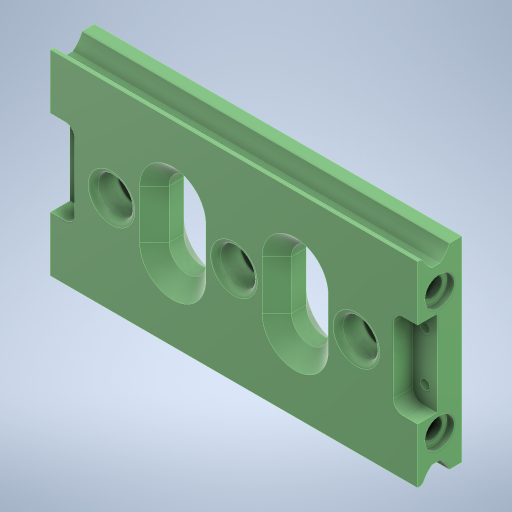
# Autodesk Inventor part: Rail-150MM
Saved by Autodesk Inventor 2023.1 (Build 271208000, 208)
## iProperties
Created: 2023-06-05
Part Number: Rail-150MM
Material: ABS Plastic
Document SubType Name: Modeling
Designer: hello
Density: 1.06 g/cm^3
Appearance: Smooth - Dark Forest Green
Mass: 267.479 g
Surface Area: 701.462 cm^2
Volume: 252.338 cm^3
Author: hello
Autodesk Inventor part; units mm, degrees
ref_plane "YZ Plane" through (0, 0, 0) normal (1, 0, 0) x (0, 1, 0)
ref_plane "XZ Plane" through (0, 0, 0) normal (0, 1, 0) x (-1, 0, 0)
ref_plane "XY Plane" through (0, 0, 0) normal (0, 0, 1) x (1, 0, 0)
sketch "Sketch1" plane through (0, 0, 0) normal (1, 0, 0) x (0, 1, 0)
  line L0 (-40, 0) -> (40, 0)
  line L1 (-40, 0) -> (-40, 5)
  line L2 (40, 0) -> (40, 5)
  line L3 (-40, 16) -> (-40, 18)
  line L4 (-40, 18) -> (40, 18)
  line L5 (40, 18) -> (40, 16)
  line L6 (0, 0) -> (0, 18) construction
  line L7 (-25, 9) -> (25, 9) construction
  circle A0 centre (-25, 9) radius 4.025
  circle A1 centre (25, 9) radius 4.025
  circle A2 centre (-40.25, 10.5) radius 5 construction
  arc A3 (-33.7571, 10.5) -> (-40, 16) centre (-44.3193, 4.8043) ccw
  arc A4 (-40, 5) -> (-33.7571, 10.5) centre (-44.3193, 16.1957) ccw
  line L8 (-40, 16) -> (-40, 5) construction
  arc A5 (40, 16) -> (33.7571, 10.5) centre (44.3193, 4.8043) ccw
  arc A6 (33.7571, 10.5) -> (40, 5) centre (44.3193, 16.1957) ccw
  line L9 (-34.8, 12.1107) -> (-34.8, 8.8893)
  line L10 (34.8, 12.1107) -> (34.8, 8.8893)
  point P0 (0, 9)
  point P1 (-40, 10.5)
  point P2 (-34.8, 10.5)
  dimension "d0" = 80
  dimension "d6" = 2
  dimension "d9" = 18
  dimension "d10" = 50
  dimension "d11" = 8.05
  dimension "d12" = 8.05
  dimension "d60" = 5
  dimension "d61" = 10
  dimension "d62" = 12
  dimension "d63" = 6.2429
  dimension "d64" = 0.25
  dimension "d65" = 12
  dimension "d66" = 12
  dimension "d67" = 6.2429
  dimension "d68" = 5.2
  constraints: 22 end point, 12 point on circle, 7 centre point, 6 midpoint, 5 horizontal alignment, 4 vertical, 3 coincident, 2 horizontal, 2 parallel, 2 tangent, 2 vertical alignment, 1 collinear, 1 equal radius, 1 perpendicular
  measures "d0" distance of L0.start L0.end
  measures "d6" distance of L3.start L3.end
  measures "d9" distance of L6.start L6.end
  measures "d10" distance of L7.start L7.end
  measures "d11" diameter of A0
  measures "d12" diameter of A1
  measures "d60" distance of L0.start L1.end
  measures "d61" diameter of A2
  measures "d62" radius of A3
  measures "d63" distance from line of A3.start L1
  measures "d64" distance of point (-40, 10.5) A2.centre
  measures "d65" radius of A5
  measures "d66" radius of A6
  measures "d67" distance from line of A5.end L2
  measures "d68" distance from line of point (-34.8, 10.5) L3
extrude "Extrusion1" add sketch "Sketch1" along normal blind 150
sketch "Sketch3" plane through (0, -40, 18) normal (0, 0, 1) x (1, 0, 0)
  line L0 (0, 80) -> (0, 0) projected
  point P0 (0, 40)
  point P1 (25, 40)
  point P2 (0, 40)
  point P3 (0, 40)
  dimension "d13" = 25
  constraints: 2 midpoint, 1 horizontal alignment
  measures "d13" distance of point (25, 40) point (0, 40)
hole "Hole1" at (25, 0, 18) direction (0, 0, -1) diameter 5.5 end through all counterbore diameter 15 counterbore depth 10 clearance for "Hex Head Cap Screw DIN EN 24017" size "M5" standard "DIN"
pattern_linear "Rectangular Pattern1" count 3 spacing 50 along (1, 0, 0) of "Hole1"
sketch "Sketch4" plane through (0, -40, 18) normal (0, 0, 1) x (1, 0, 0)
  line L0 (0, 57.5) -> (6, 57.5)
  line L1 (10, 53.5) -> (10, 26.5)
  line L2 (6, 22.5) -> (0, 22.5)
  line L3 (0, 22.5) -> (0, 57.5)
  line L4 (0, 80) -> (0, 0) construction
  arc A0 (10, 53.5) -> (6, 57.5) centre (6, 53.5) ccw
  arc A1 (6, 22.5) -> (10, 26.5) centre (6, 26.5) ccw
  line L5 (144, 57.5) -> (150, 57.5)
  line L6 (150, 57.5) -> (150, 22.5)
  line L7 (150, 22.5) -> (144, 22.5)
  line L8 (140, 26.5) -> (140, 53.5)
  line L9 (150, 80) -> (150, 0) construction
  arc A2 (144, 57.5) -> (140, 53.5) centre (144, 53.5) ccw
  arc A3 (140, 26.5) -> (144, 22.5) centre (144, 26.5) ccw
  point P0 (0, 40)
  point P1 (10, 22.5)
  point P2 (10, 57.5)
  point P3 (0, 40)
  point P4 (140, 22.5)
  point P5 (150, 40)
  dimension "d24" = 10
  dimension "d25" = 35
  dimension "d26" = 4
  dimension "d27" = 10
  dimension "d28" = 4
  constraints: 16 end point, 8 point on circle, 8 tangent, 6 point on line, 5 parallel, 4 centre point, 4 midpoint, 2 equal radius, 2 horizontal, 2 perpendicular
  measures "d24" distance of point (10, 22.5) L2.end
  measures "d25" distance of point (10, 57.5) point (10, 22.5)
  measures "d26" radius of A0
  measures "d27" distance of L6.end point (140, 22.5)
  measures "d28" radius of A2
extrude "Extrusion2" cut sketch "Sketch4" against normal blind 8
sketch "Sketch5" plane through (0, -40, 10) normal (0, 0, 1) x (1, 0, 0)
  line L0 (0, 57.5) -> (6, 57.5) projected
  line L1 (0, 22.5) -> (0, 57.5) projected
  line L2 (6, 22.5) -> (0, 22.5) projected
  arc A0 (6, 22.5) -> (10, 26.5) centre (6, 26.5) ccw projected
  line L3 (10, 53.5) -> (10, 26.5) projected
  arc A1 (10, 53.5) -> (6, 57.5) centre (6, 53.5) ccw projected
  arc A2 (144, 57.5) -> (140, 53.5) centre (144, 53.5) ccw projected
  line L4 (140, 26.5) -> (140, 53.5) projected
  arc A3 (140, 26.5) -> (144, 22.5) centre (144, 26.5) ccw projected
  line L5 (150, 57.5) -> (150, 22.5) projected
  line L6 (10, 53.5) -> (10, 26.5) projected
  line L7 (10, 40) -> (0, 40)
  line L8 (5, 50) -> (5, 30)
  line L9 (140, 26.5) -> (140, 53.5) projected
  line L10 (140, 40) -> (150, 40)
  line L11 (145, 50) -> (145, 30)
  line L12 (150, 22.5) -> (144, 22.5) projected
  line L13 (144, 57.5) -> (150, 57.5) projected
  point P0 (5, 40)
  point P1 (145, 40)
  dimension "d31" = 20
  constraints: 8 end point, 7 midpoint, 4 coincident, 2 vertical, 1 horizontal, 1 horizontal alignment
  measures "d31" distance of L8.start L8.end
hole "Hole2" at (5, 10, 10) at (5, -10, 10) at (145, 10, 10) at (145, -10, 10) direction (0, 0, -1) diameter 4 depth 5
sketch "Sketch6" plane through (0, 40, 18) normal (0, 0, 1) x (1, 0, 0)
  line L0 (50, -50) -> (50, -30) construction
  line L1 (150, -19.025) -> (0, -19.025) projected
  line L2 (57.5, -50) -> (57.5, -30)
  line L3 (42.5, -30) -> (42.5, -50)
  arc A0 (42.5, -50) -> (57.5, -50) centre (50, -50) ccw
  arc A1 (57.5, -30) -> (42.5, -30) centre (50, -30) ccw
  circle A2 centre (75, -40) radius 2.75 projected
  circle A3 centre (25, -40) radius 2.75 projected
  circle A4 centre (25, -40) radius 2.75 projected
  line L4 (25, -40) -> (75, -40)
  arc A5 (107.5, -30) -> (92.5, -30) centre (100, -30) ccw
  line L5 (107.5, -50) -> (107.5, -30)
  line L6 (92.5, -30) -> (92.5, -50)
  arc A6 (92.5, -50) -> (107.5, -50) centre (100, -50) ccw
  point P0 (0, -40)
  point P1 (50, -40)
  point P2 (50, -40)
  dimension "d39" = 10
  dimension "d40" = 15
  dimension "d43" = 50
  constraints: 14 end point, 8 point on circle, 4 centre point, 4 tangent, 2 horizontal, 2 midpoint, 1 coincident, 1 parallel, 1 perpendicular, 10 other
  measures "d39" distance of point (50, -40) L0.end
  measures "d40" diameter of A1
  measures "d43" distance of L0.end A5.centre
extrude "Extrusion3" cut sketch "Sketch6" against normal through all contours A0 L3 L4 L2 | L4 L3 A1 L2 | L5 A6 L6 A5
chamfer "Chamfer1" distance 6 angle 45 16 edges at (50, 17.5, 18) (57.5, 0, 18) (50, -17.5, 18) (42.5, 0, 18) (100, 17.5, 18) (107.5, 0, 18) (100, -17.5, 18) (92.5, 0, 18) (100, 17.5, 0) (92.5, 0, 0) (100, -17.5, 0) (107.5, 0, 0) (42.5, 0, 0) (50, -17.5, 0) (57.5, 0, 0) (50, 17.5, 0)
sketch "Sketch7" plane through (0, 0, 0) normal (-1, 0, 0) x (0, 0, 1)
  circle A0 centre (9, 25) radius 4.025 projected
  circle A1 centre (9, -25) radius 4.025 projected
  circle A2 centre (9, 25) radius 6
  circle A3 centre (9, -25) radius 6
  point P0 (0, 0)
  dimension "d53" = 12
  dimension "d54" = 12
  constraints: 2 centre point, 2 coincident
  measures "d53" diameter of A2
  measures "d54" diameter of A3
extrude "Extrusion4" cut sketch "Sketch7" against normal blind 3
sketch "Sketch8" plane through (150, 0, 0) normal (1, 0, 0) x (0, 0, -1)
  circle A0 centre (-9, -25) radius 6 projected
  circle A1 centre (-9, 25) radius 6 projected
  point P0 (0, 0)
extrude "Extrusion5" cut sketch "Sketch8" against normal blind 3
fillet "Fillet1" radius 2 3 edges at (75, 7.5, 18) (25, 7.5, 18) (125, 7.5, 18)
fillet "Fillet3" radius 2 2 edges at (75, 40, 16) (75, -40, 16)
equation "\"d12\" = d11"
equation "\"d67\" = d63"
body "Solid1"
